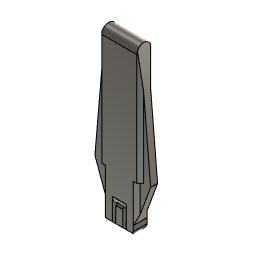
EvricsTopV1 v1 (Autodesk Fusion 360 design; units mm, degrees)
Autodesk Fusion 360 part; units mm, degrees
sketch "Sketch1" plane through (0, 0, 0) normal (0, 1, 0) x (1, 0, 0)
  line L0 (0, 0) -> (-12.7, 0)
  line L1 (-12.7, 0) -> (-12.7, -86.518)
  line L2 (-12.7, -86.518) -> (0, -86.518)
  line L3 (0, -86.518) -> (0, 0)
  line L4 (0, 0) -> (-10.16, 0)
  line L5 (-10.16, 0) -> (-10.16, 35.56)
  line L6 (-10.16, 35.56) -> (-5.08, 35.56)
  line L7 (0, 22.86) -> (0, 0)
  line L8 (-12.7, -86.518) -> (-20.32, 0)
  line L9 (-20.32, 0) -> (-10.16, 27.94)
  line L10 (12.7, 0) -> (12.7, -86.518)
  line L11 (12.7, -86.518) -> (0, -86.518)
  line L12 (12.7, -86.518) -> (20.32, 0)
  line L13 (20.32, 0) -> (10.16, 27.94)
  line L14 (10.16, 0) -> (10.16, 35.56)
  line L15 (0, 0) -> (12.7, 0)
  line L16 (10.16, 35.56) -> (5.08, 35.56)
  line L17 (5.08, 35.56) -> (5.08, 22.86)
  line L18 (5.08, 22.86) -> (-5.08, 22.86)
  line L19 (-5.08, 22.86) -> (-5.08, 35.56)
  dimension "d1" = 12.7
  constraint horizontal L0
  constraint vertical L1
  constraint horizontal L2
  constraint vertical L3
  constraint coincident L0.start L3.end
  constraint horizontal L4
  constraint vertical L5
  constraint horizontal L6
  constraint vertical L7
  constraint coincident L5 L9.end
  constraint symmetric L0.start L7 L3.end
  constraint symmetric L0.end L7 L10.start
  constraint symmetric L1.end L7 L10.end
  constraint symmetric L2.end L7 L3.start
  constraint symmetric L4.end L7 L14.start
  constraint symmetric L5.end L7 L14.end
  constraint symmetric L7 L8.end L12.end
  constraint symmetric L7 L9.end L13.end
  constraint vertical L17
  constraint horizontal L18
  constraint vertical L19
  constraint coincident L18 L7.start
  measures "d1" distance of L0.start L0.end
extrude "Extrude2" add sketch "Sketch1" along normal mid plane 10.16 contours L0 L1 L2 L3 L4 | L3 L10 L11 L15 | L0 L4 L5 L6 L7 L18 L19 | L7 L14 L15 L16 L17 L18 makes body 1
extrude "Extrude1" add sketch "Sketch1" along normal blind 7.62 separate body contours L0 L1 L2 L3 L4 | L3 L10 L11 L15 | L0 L4 L5 L6 L7 L18 L19 | L7 L14 L15 L16 L17 L18 makes body 2
extrude "Extrude3" add sketch "Sketch1" along normal mid plane 5.08 contours L0 L1 L5 L8 L9 | L10 L12 L13 L14 L15 bodies 1 2
chamfer "Chamfer1" distance 2.54 angle 45 8 edges at (12.7, 2.54, 43.259) (10.16, 2.54, -13.97) (-12.7, 2.54, 43.259) (-10.16, 2.54, -13.97) (-12.7, -2.54, 43.259) (-10.16, -2.54, -13.97) (12.7, -2.54, 43.259) (10.16, -2.54, -13.97) on bodies 1
extrude "Extrude4" cut 1 faces at (3.3867, 7.62, 57.6787) along direction (0, -1, 0) blind 2.54 on bodies 1 bodies 1
fillet "Fillet1" radius 5.08 2 edges at (0, -5.08, 86.518) (0, 5.08, 86.518) on bodies 1
chamfer "Chamfer2" distance 2.54 angle 45 4 edges at (-7.62, 5.08, -35.56) (7.62, 5.08, -35.56) (7.62, -5.08, -35.56) (-7.62, -5.08, -35.56) on bodies 1
fillet "Fillet2" radius 6.35 2 edges at (0, 5.08, -22.86) (0, -5.08, -22.86) on bodies 1
ref_plane "WorkPlane1" through (0, 5.08, 24.209) normal (0, 1, 0) x (0, 0, 1)
sketch "Sketch2" plane through (0, 5.08, 24.209) normal (0, 1, 0) x (1, 0, 0)
  line L0 (7.62, -48.26) -> (0, -48.26)
  line L1 (-7.62, -48.26) -> (0, -48.26)
  line L2 (7.62, -48.26) -> (-7.62, -48.26)
  line L3 (-7.62, -48.26) -> (-7.62, -40.64)
  line L4 (-7.62, -40.64) -> (7.62, -40.64)
  line L5 (7.62, -40.64) -> (7.62, -48.26)
  line L6 (7.62, -40.64) -> (-7.62, -40.64)
  line L7 (-7.62, -35.56) -> (7.62, -35.56)
  line L8 (7.62, -35.56) -> (-7.62, -35.56)
  line L9 (-7.62, -35.56) -> (-7.62, -27.94)
  line L10 (-7.62, -27.94) -> (7.62, -27.94)
  line L11 (7.62, -27.94) -> (7.62, -35.56)
  line L12 (7.62, -27.94) -> (-7.62, -27.94)
  line L13 (-7.62, -22.86) -> (7.62, -22.86)
  line L14 (7.62, -22.86) -> (-7.62, -22.86)
  line L15 (-7.62, -22.86) -> (-7.62, -15.24)
  line L16 (-7.62, -15.24) -> (7.62, -15.24)
  line L17 (7.62, -15.24) -> (7.62, -22.86)
  line L18 (7.62, -15.24) -> (-7.62, -15.24)
  line L19 (-7.62, -10.16) -> (7.62, -10.16)
  line L20 (7.62, -10.16) -> (-7.62, -10.16)
  line L21 (-7.62, -10.16) -> (-7.62, -2.54)
  line L22 (-7.62, -2.54) -> (7.62, -2.54)
  line L23 (7.62, -2.54) -> (7.62, -10.16)
  line L24 (7.62, -2.54) -> (-7.62, -2.54)
  line L25 (-7.62, 2.54) -> (7.62, 2.54)
  line L26 (7.62, 2.54) -> (-7.62, 2.54)
  line L27 (-7.62, 2.54) -> (-7.62, 10.16)
  line L28 (-7.62, 10.16) -> (7.62, 10.16)
  line L29 (7.62, 10.16) -> (7.62, 2.54)
  line L30 (7.62, 10.16) -> (-7.62, 10.16)
  line L31 (7.62, -40.64) -> (7.62, -48.26)
  line L32 (-7.62, -40.64) -> (-7.62, -48.26)
  line L33 (7.62, -27.94) -> (7.62, -35.56)
  line L34 (-7.62, -27.94) -> (-7.62, -35.56)
  line L35 (7.62, -2.54) -> (7.62, -10.16)
  line L36 (7.62, -15.24) -> (7.62, -22.86)
  line L37 (-7.62, -2.54) -> (-7.62, -10.16)
  line L38 (-7.62, -15.24) -> (-7.62, -22.86)
  line L39 (7.62, 10.16) -> (7.62, 2.54)
  line L40 (-7.62, 2.54) -> (-7.62, 10.16)
  line L41 (2.54, -48.26) -> (0, -48.26)
  line L42 (0, -48.26) -> (-2.54, -48.26)
  line L43 (-2.54, 0) -> (-2.54, 2.54)
  line L44 (-2.54, 10.16) -> (2.54, 10.16)
  line L45 (2.54, 2.54) -> (2.54, 0)
  line L46 (2.54, 0) -> (2.54, -2.54)
  line L47 (-2.54, -2.54) -> (-2.54, 0)
  line L48 (2.54, -35.56) -> (2.54, -40.64)
  line L49 (-2.54, -40.64) -> (-2.54, -35.56)
  line L50 (2.54, -10.16) -> (2.54, -15.24)
  line L51 (2.54, -22.86) -> (2.54, -27.94)
  line L52 (0, -27.94) -> (0, -22.86)
  line L53 (0, -15.24) -> (0, -10.16)
  line L54 (-2.54, -27.94) -> (-2.54, -22.86)
  line L55 (-2.54, -15.24) -> (-2.54, -10.16)
  line L56 (0, -22.86) -> (0, -27.94)
  line L57 (0, -10.16) -> (0, -15.24)
  constraint vertical L35
  constraint horizontal L0
  constraint vertical L37
  constraint horizontal L1
  constraint vertical L40
  constraint horizontal L2
  constraint vertical L3
  constraint horizontal L4
  constraint vertical L5
  constraint coincident L3.end L37
  constraint horizontal L6
  constraint horizontal L7
  constraint horizontal L8
  constraint vertical L9
  constraint horizontal L10
  constraint vertical L11
  constraint coincident L9.end L37
  constraint horizontal L12
  constraint horizontal L13
  constraint horizontal L14
  constraint vertical L15
  constraint horizontal L16
  constraint vertical L17
  constraint horizontal L18
  constraint horizontal L19
  constraint horizontal L20
  constraint vertical L21
  constraint horizontal L22
  constraint vertical L23
  constraint horizontal L24
  constraint horizontal L25
  constraint horizontal L26
  constraint vertical L27
  constraint horizontal L28
  constraint vertical L29
  constraint horizontal L30
  constraint collinear L31 L35
  constraint collinear L32 L37
  constraint collinear L33 L35
  constraint collinear L34 L37
  constraint collinear L35 L36
  constraint collinear L37 L38
  constraint vertical L46
  constraint horizontal L41
  constraint coincident L2 L41.start
  constraint horizontal L42
  constraint vertical L49
  constraint vertical L43
  constraint horizontal L44
  constraint vertical L45
  constraint coincident L30 L44.start
  constraint coincident L25 L43.end
  constraint coincident L25 L45.start
  constraint coincident L22 L46.end
  constraint coincident L19 L50.start
  constraint collinear L46 L50
  constraint coincident L19 L55.end
  constraint coincident L22 L47.start
  constraint collinear L47 L49
  constraint coincident L19 L53.end
  constraint coincident L4 L49.start
  constraint coincident L4 L48.end
  constraint coincident L10 L51.end
  constraint coincident L7 L48.start
  constraint collinear L48 L50
  constraint coincident L10 L52.start
  constraint coincident L7 L49.end
  constraint coincident L10 L54.start
  constraint collinear L49 L54
  constraint coincident L16 L50.end
  constraint coincident L13 L51.start
  constraint collinear L50 L51
  constraint coincident L13 L52.end
  constraint coincident L16 L53.start
  constraint collinear L52 L53
  constraint coincident L13 L54.end
  constraint coincident L16 L55.start
  constraint collinear L54 L55
extrude "Extrude5" add sketch "Sketch2" along normal blind 2.54 contours L0 L1 L2 L3 L4 L5 L6 L31 L32 L41 L42 | L7 L8 L9 L10 L11 L12 L33 L34 | L13 L14 L15 L16 L17 L18 L36 L38 | L19 L20 L21 L22 L23 L24 L35 L37 | L25 L26 L27 L28 L29 L30 L39 L40 L44 bodies 1
extrude "Extrude6" add sketch "Sketch2" along normal blind 1.905 contours L4 L6 L7 L8 L48 L49 | L10 L12 L13 L14 L51 L52 L56 | L10 L12 L13 L14 L52 L54 L56 | L16 L18 L19 L20 L50 L53 L57 | L16 L18 L19 L20 L53 L55 L57 | L22 L24 L25 L26 L43 L45 L46 L47 bodies 1
chamfer "Chamfer3" distance 1.27 angle 45 8 edges at (2.54, 6.985, 62.309) (-2.54, 6.985, 62.309) (2.54, 6.985, 49.609) (-2.54, 6.985, 49.609) (2.54, 6.985, 36.909) (-2.54, 6.985, 36.909) (2.54, 6.985, 24.209) (-2.54, 6.985, 24.209) on bodies 1
fillet "Fillet3" radius 10.16 10 edges at (7.62, 7.62, 17.859) (-7.62, 7.62, 17.859) (7.62, 7.62, 30.559) (-7.62, 7.62, 30.559) (7.62, 7.62, 43.259) (7.62, 7.62, 55.959) (7.62, 7.62, 68.659) (-7.62, 7.62, 68.659) (-7.62, 7.62, 55.959) (-7.62, 7.62, 43.259) on bodies 1
sketch "Sketch3" plane through (0, 5.08, 0) normal (0, 1, 0) x (-1, 0, 0)
  line L0 (-2.54, 21.669) -> (-2.54, 26.749)
  line L1 (-2.54, 26.749) -> (-7.62, 26.749)
  line L2 (-7.62, 26.749) -> (-7.62, 34.369)
  line L3 (-7.62, 34.369) -> (-2.54, 34.369)
  line L4 (-2.54, 34.369) -> (-2.54, 39.449)
  line L5 (-2.54, 39.449) -> (-7.62, 39.449)
  line L6 (-7.62, 39.449) -> (-7.62, 47.069)
  line L7 (-7.62, 47.069) -> (-2.54, 47.069)
  line L8 (-2.54, 47.069) -> (-2.54, 52.149)
  line L9 (-2.54, 52.149) -> (-7.62, 52.149)
  line L10 (-7.62, 52.149) -> (-7.62, 59.769)
  line L11 (-7.62, 59.769) -> (-2.54, 59.769)
  line L12 (-2.54, 59.769) -> (-2.54, 64.849)
  line L13 (-2.54, 64.849) -> (-7.62, 64.849)
  line L14 (-7.62, 64.849) -> (-7.62, 72.469)
  line L15 (-7.62, 72.469) -> (7.62, 72.469)
  line L16 (7.62, 72.469) -> (7.62, 64.849)
  line L17 (7.62, 64.849) -> (2.54, 64.849)
  line L18 (2.54, 64.849) -> (2.54, 59.769)
  line L19 (2.54, 59.769) -> (7.62, 59.769)
  line L20 (7.62, 59.769) -> (7.62, 52.149)
  line L21 (7.62, 52.149) -> (2.54, 52.149)
  line L22 (2.54, 52.149) -> (2.54, 47.069)
  line L23 (2.54, 47.069) -> (7.62, 47.069)
  line L24 (7.62, 47.069) -> (7.62, 39.449)
  line L25 (7.62, 39.449) -> (2.54, 39.449)
  line L26 (2.54, 39.449) -> (2.54, 34.369)
  line L27 (2.54, 34.369) -> (7.62, 34.369)
  line L28 (7.62, 34.369) -> (7.62, 26.749)
  line L29 (7.62, 26.749) -> (2.54, 26.749)
  line L30 (2.54, 26.749) -> (2.54, 21.669)
  line L31 (2.54, 21.669) -> (7.62, 21.669)
  line L32 (7.62, 21.669) -> (7.62, 14.049)
  line L33 (7.62, 14.049) -> (-7.62, 14.049)
  line L34 (-7.62, 14.049) -> (-7.62, 21.669)
  line L35 (-7.62, 21.669) -> (-2.54, 21.669)
  line L36 (-5.08, -33.02) -> (-5.08, -16.51)
  line L37 (-5.08, -16.51) -> (5.08, -16.51)
  line L38 (5.08, -16.51) -> (5.08, -33.02)
  line L39 (5.08, -33.02) -> (10.16, -33.02)
  line L40 (10.16, -33.02) -> (10.16, -27.94)
  line L41 (10.16, -27.94) -> (10.16, 0)
  line L42 (10.16, 0) -> (12.7, 0)
  line L43 (12.7, 0) -> (12.7, 81.438)
  line L44 (12.7, 81.438) -> (-12.7, 81.438)
  line L45 (-12.7, 81.438) -> (-12.7, 0)
  line L46 (-12.7, 0) -> (-10.16, 0)
  line L47 (-10.16, 0) -> (-10.16, -27.94)
  line L48 (-10.16, -27.94) -> (-10.16, -33.02)
  line L49 (-10.16, -33.02) -> (-5.08, -33.02)
  circle A0 centre (0, 0) radius 8.89
  line L50 (-5.08, 0) -> (0, 8.89)
  line L51 (0, 8.89) -> (5.08, 0)
  line L52 (5.08, 0) -> (2.54, -8.5194)
  line L53 (-2.54, -8.5194) -> (-5.08, 0)
  line L54 (2.54, -8.5194) -> (-2.54, -8.5194)
  dimension "d24" = 17.78
  constraint coincident A0.centre origin
  constraint coincident A0 L50.end
  constraint coincident A0 L52.end
  constraint coincident A0 L53.start
  constraint horizontal L54
  measures "d24" diameter of A0
extrude "Extrude7" add sketch "Sketch3" along normal blind 2.54 contours L50 L51 L52 L53 L54 bodies 1
extrude "Extrude8" add sketch "Sketch3" along normal blind 1.905 contours A0 L51 L52 | A0 L50 L53 bodies 1
fillet "Fillet4" radius 20.32 1 edges at (0, 7.62, -8.5194) on bodies 1
sketch "Sketch4" plane through (0, 0, 0) normal (0, 1, 0) x (1, 0, 0)
  line L0 (0, 22.86) -> (2.54, 22.86)
  line L1 (2.54, 22.86) -> (2.54, 33.02)
  line L2 (2.54, 33.02) -> (0, 33.02)
  line L3 (0, 33.02) -> (0, 22.86)
  line L4 (-2.54, 33.02) -> (0, 33.02)
  line L5 (0, 33.02) -> (0, 22.86)
  line L6 (0, 22.86) -> (-2.54, 22.86)
  line L7 (-2.54, 22.86) -> (-2.54, 33.02)
  point P0 (0, 22.86)
  constraint horizontal L0
  constraint vertical L1
  constraint horizontal L2
  constraint vertical L3
  constraint coincident P0 L0.start
  constraint horizontal L4
  constraint vertical L5
  constraint horizontal L6
  constraint vertical L7
extrude "Extrude9" add sketch "Sketch4" along normal mid plane 10.16 separate body makes body 3
extrude "Extrude10" add 1 faces at (0.8467, -1.6933, -33.02) along direction (0, 0, -1) blind 2.54 on bodies 3 bodies 3
sketch "Sketch5" plane through (-2.54, 0, 0) normal (-1, 0, 0) x (0, -1, 0)
  line L0 (5.08, -22.86) -> (-5.08, -22.86)
  line L1 (-5.08, -22.86) -> (-5.08, -35.56)
  line L2 (-5.08, -35.56) -> (5.08, -35.56)
  line L3 (5.08, -35.56) -> (5.08, -22.86)
  line L4 (0, -22.86) -> (0, -33.02)
  line L5 (0, -35.56) -> (0, -27.94) construction
  line L6 (0, -35.56) -> (0, -31.75) construction
  circle A0 centre (0, -31.75) radius 2.8575
  dimension "d35" = 7.62
  dimension "d36" = 3.81
  dimension "d37" = 5.715
  constraint midpoint L2 L5.start
  constraint midpoint L4 L5.end
  constraint perpendicular L2 L6
  constraint coincident L6.end A0.centre
  measures "d35" distance of L5.start L5.end
  measures "d36" distance of L5.start L6.end
  measures "d37" diameter of A0
extrude "Extrude11" cut sketch "Sketch5" along normal blind 5.08 and the other way blind 10.16 contours A0 bodies 1 3
chamfer "Chamfer4" distance 2.54 angle 45 2 edges at (0, 5.08, -35.56) (0, -5.08, -35.56) on bodies 3
fillet "Fillet5" radius 3.81 2 edges at (-10.16, 0, -35.56) (10.16, 0, -35.56) on bodies 1
extrude "Extrude12" add 1 faces at (-0.8467, -1.6933, -22.86) along direction (0, 0, 1) blind 1.27 on bodies 3 bodies 3 1
fillet "Fillet6" radius 1.27 2 edges at (0, 2.54, -21.59) (0, -3.1596, -21.59) on bodies 3
